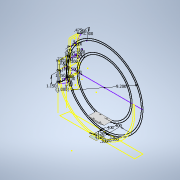
# Autodesk Inventor part: headband buffer
Saved by Autodesk Inventor 2022 (Build 260153000, 153)
## iProperties
Created: 2021-04-08
Part Number: headband buffer
Material: Generic
Document SubType Name: Modeling
Designer: chris
Density: 1 g/cm^3
Appearance: Default
Author: chris
Autodesk Inventor part; units mm, degrees
ref_plane "YZ Plane" through (0, 0, 0) normal (1, 0, 0) x (0, 1, 0)
ref_plane "XZ Plane" through (0, 0, 0) normal (0, 1, 0) x (-1, 0, 0)
ref_plane "XY Plane" through (0, 0, 0) normal (0, 0, 1) x (1, 0, 0)
sketch "Sketch1" plane through (0, 0, 0) normal (0, 0, 1) x (1, 0, 0)
  circle A0 centre (0, 0) radius 116.84
  circle A1 centre (0, 0) radius 111.76
  line L0 (-116.84, 0) -> (116.84, 0)
  circle A2 centre (0, 0) radius 78.74
  circle A3 centre (0, 0) radius 83.82
  point P0 (111.76, 0)
  point P1 (-111.76, 0)
  point P2 (-83.82, 0)
  point P3 (83.82, 0)
  point P4 (78.74, 0)
  point P5 (-78.74, 0)
  dimension "d0" = 233.68
  dimension "d1" = 5.08
  dimension "d45" = 38.1
  dimension "d46" = 5.08
  constraints: 4 centre point, 2 end point, 2 point on circle, 1 coincident, 1 horizontal
  measures "d0" diameter of A0
  measures "d1" radial gap between concentric circles of A0 A1
  measures "d45" radial gap between concentric circles of A0 A2
  measures "d46" radial gap between concentric circles of A2 A3
extrude "Extrusion1" add sketch "Sketch1" along normal blind 25.4 contours A0 L0 A1 picked at (7.308, -113.0578)
sketch "Sketch2" plane through (-116.84, 0, 0) normal (0, 1, 0) x (1, 0, 0)
  line L0 (5.08, 0) -> (0, 0) projected
  line L1 (0, 0) -> (0, -25.4) projected
  line L2 (5.08, -25.4) -> (0, -25.4) projected
  line L3 (5.08, 0) -> (5.08, -25.4) projected
  line L4 (233.68, 0) -> (228.6, 0) projected
  line L5 (228.6, 0) -> (228.6, -25.4) projected
  line L6 (233.68, -25.4) -> (228.6, -25.4) projected
  line L7 (233.68, 0) -> (233.68, -25.4) projected
  point P0 (116.84, 0)
extrude "Extrusion2" add sketch "Sketch2" along normal blind 25.4
sketch "Sketch3" plane through (-116.84, 0, 25.4) normal (-1, 0, 0) x (0, 0, 1)
  line L0 (-25.4, 0) -> (0, 0) projected
  line L1 (0, 0) -> (0, -34.29)
  line L2 (0, 0) -> (0, -111.76) projected
  line L3 (0, -34.29) -> (-25.4, -34.29)
  line L4 (-25.4, 0) -> (-25.4, -111.76) projected
  line L5 (-25.4, -34.29) -> (-25.4, 0)
  circle A0 centre (-5.7404, -2.54) radius 1.524
  circle A1 centre (-5.7404, -31.75) radius 1.524
  circle A2 centre (-19.6538, -2.54) radius 1.524
  circle A3 centre (-19.6538, -31.75) radius 1.524
  dimension "d6" = 34.29
  dimension "d7" = 3.048
  dimension "d8" = 3.048
  dimension "d9" = 3.048
  dimension "d10" = 3.048
  dimension "d11" = 29.21
  dimension "d12" = 2.54
  dimension "d13" = 5.7404
  constraints: 6 end point, 4 centre point, 2 horizontal alignment, 2 perpendicular, 2 point on line, 2 vertical alignment
  measures "d6" distance of L0.end L1.end
  measures "d7" diameter of A0
  measures "d8" diameter of A1
  measures "d9" diameter of A2
  measures "d10" diameter of A3
  measures "d11" distance of A1.centre A0.centre
  measures "d12" distance from line of L3 A1.centre
  measures "d13" distance from line of L1 A1.centre
extrude "Extrusion3" add sketch "Sketch3" against normal up to surface round surface about axis through (0, 0, 0) along (0, 0, 1) radius 116.84 far side no
extrude "Extrusion4" cut sketch "Sketch3" against normal blind 38.1 contours A0 | A1 | A2 | A3
sketch "Sketch4" plane through (-116.84, 25.4, 0) normal (-1, 0, 0) x (0, 0, 1)
  circle A0 centre (5.7462, -57.15) radius 1.524 projected
  circle A1 centre (5.7462, -27.94) radius 1.524 projected
  circle A2 centre (19.6596, -57.15) radius 1.524 projected
  circle A3 centre (19.6596, -27.94) radius 1.524 projected
  line L0 (25.4, -59.69) -> (25.4, 0) projected
  line L1 (0, 0) -> (25.4, 0) projected
  line L2 (0, -59.69) -> (0, 0) projected
  line L3 (0, -59.69) -> (25.4, -59.69) projected
  arc A4 (-7.874, -68.071) -> (0, -59.69) centre (-15.4136, -53.0981) ccw
  line L4 (-7.874, -68.071) -> (0, -71.373)
  line L5 (0, -25.4) -> (0, -137.16) projected
  line L6 (0, -71.373) -> (25.4, -59.69)
  arc A5 (0, -25.4) -> (-12.065, -6.604) centre (-32.1829, -32.7878) ccw
  line L7 (-12.065, -6.604) -> (0, 0)
  dimension "d22" = 16.764
  dimension "d23" = 33.02
  dimension "d24" = 6.604
  dimension "d25" = 12.065
  dimension "d26" = 7.874
  dimension "d27" = 3.302
  dimension "d28" = 25.4
  constraints: 6 end point, 4 point on circle, 2 centre point, 1 point on line
  measures "d22" radius of A4
  measures "d23" radius of A5
  measures "d24" vertical distance of L7.start L1.start
  measures "d25" horizontal distance of L1.start L7.start
  measures "d26" horizontal distance of L4.end L4.start
  measures "d27" vertical distance of L4.end L4.start
  measures "d28" horizontal distance of L0.start L4.end
extrude "Extrusion5" add sketch "Sketch4" against normal up to surface contours L6 L5 L3 | L5 L4 A4 round surface about axis through (0, 0, 0) along (0, 0, 1) radius 116.84 far side no
extrude "Extrusion6" add sketch "Sketch4" against normal up to surface (5.08 mm away) contours L2 A5 L7
sketch "Sketch5" plane through (116.84, 0, 0) normal (1, 0, 0) x (0, 0, -1)
  line L0 (0, 0) -> (-25.4, 0) projected
  line L1 (0, 0) -> (0, 25.4) projected
  line L2 (-25.4, 25.4) -> (0, 25.4) projected
  line L3 (-25.4, 0) -> (-25.4, 25.4) projected
  circle A0 centre (-12.7, 4.445) radius 1.524
  circle A1 centre (-12.7, 20.955) radius 1.524
  dimension "d29" = 3.048
  dimension "d30" = 3.048
  dimension "d31" = 4.445
  dimension "d32" = 4.445
  constraints: 2 centre point
  measures "d29" diameter of A0
  measures "d30" diameter of A1
  measures "d31" distance from line of L2 A1.centre
  measures "d32" distance from line of L0 A0.centre
extrude "Extrusion7" cut sketch "Sketch5" against normal blind 38.1 contours A0 | A1
sketch "Sketch6" plane through (0, 0, 25.4) normal (0, 0, 1) x (1, 0, 0)
  arc A0 (-111.76, 0) -> (111.76, 0) centre (0, 0) ccw projected
  line L0 (-111.76, 0) -> (-111.76, 25.4) projected
  line L1 (-116.84, 25.4) -> (-111.76, 25.4) projected
  line L2 (-116.84, -34.29) -> (-116.84, 25.4) projected
  line L3 (-116.84, -34.29) -> (-111.695, -34.29) projected
  arc A1 (-111.695, -34.29) -> (116.84, 0) centre (0, 0) ccw projected
  line L4 (116.84, 0) -> (116.84, 25.4) projected
  line L5 (111.76, 25.4) -> (116.84, 25.4) projected
  line L6 (111.76, 0) -> (111.76, 25.4) projected
  arc A2 (-107.4154, -45.973) -> (116.84, 0) centre (0, 0) ccw projected
  point P0 (0, -116.84)
  constraints: 1 point on circle
ref_plane "Work Plane1" through (0, -116.84, 25.4) normal (0, -1, 0) x (1, 0, 0)
sketch "Sketch7" plane through (0, -116.84, 25.4) normal (0, -1, 0) x (1, 0, 0)
  ellipse E0 centre (0, 74.5502) end of major axis (0, 328.573) minor radius 116.84 (-111.695, 0) -> (-107.4154, -25.4) ccw projected
  line L0 (-107.4154, -25.4) -> (116.84, -25.4) projected
  line L1 (116.84, -25.4) -> (116.84, 0) projected
  line L2 (-111.695, 0) -> (116.84, 0) projected
  circle A0 centre (10.16, -2.54) radius 1.524
  circle A1 centre (-10.16, -2.54) radius 1.524
  circle A2 centre (-10.16, -22.86) radius 1.524
  circle A3 centre (10.16, -22.86) radius 1.524
  point P0 (0, -25.4)
  dimension "d35" = 3.048
  dimension "d36" = 3.048
  dimension "d37" = 10.16
  dimension "d38" = 10.16
  dimension "d39" = 2.54
  dimension "d40" = 3.048
  dimension "d41" = 3.048
  dimension "d42" = 2.54
  constraints: 4 centre point, 2 horizontal alignment, 2 vertical alignment, 1 other
  measures "d35" diameter of A0
  measures "d36" diameter of A1
  measures "d37" horizontal distance of point (0, -25.4) A0.centre
  measures "d38" horizontal distance of point (0, -25.4) A1.centre
  measures "d39" distance from line of L2 A1.centre
  measures "d40" diameter of A2
  measures "d41" diameter of A3
  measures "d42" distance from line of L0 A3.centre
extrude "Extrusion8" cut sketch "Sketch7" against normal blind 38.1 contours A0 | A1 | A2 | A3
extrude "Extrusion9" add sketch "Sketch1" along normal blind 25.4 contours A3 L0 A2 picked at (6.1938, -80.0321)
sketch "Sketch8" plane through (78.74, 0, 0) normal (0, 1, 0) x (1, 0, 0)
  line L0 (5.08, 0) -> (0, 0) projected
  line L1 (0, 0) -> (0, -25.4) projected
  line L2 (5.08, -25.4) -> (0, -25.4) projected
  line L3 (5.08, 0) -> (5.08, -25.4) projected
  line L4 (-157.48, 0) -> (-162.56, 0) projected
  line L5 (-162.56, 0) -> (-162.56, -25.4) projected
  line L6 (-157.48, -25.4) -> (-162.56, -25.4) projected
  line L7 (-157.48, 0) -> (-157.48, -25.4) projected
  point P0 (-78.74, 0)
extrude "Extrusion10" add sketch "Sketch8" along normal blind 101.6
sketch "Sketch9" plane through (-83.82, 0, 25.4) normal (-1, 0, 0) x (0, 0, 1)
  point P0 (-25.4, 0)
sketch "Sketch10" plane through (-83.82, 0, 25.4) normal (-1, 0, 0) x (0, 0, 1)
  line L0 (-25.4, 0) -> (0, 0) projected
  line L1 (0, 0) -> (0, 101.6) projected
  line L2 (-25.4, 101.6) -> (0, 101.6) projected
  line L3 (-25.4, 0) -> (-25.4, 101.6) projected
  line L4 (-25.4, 0) -> (-25.4, 101.6) projected
  line L5 (-25.4, 101.6) -> (-37.465, 94.996)
  arc A0 (-25.4, 81.4487) -> (-37.465, 94.996) centre (-55.1426, 67.1065) ccw
  line L6 (-25.4, 33.6843) -> (-33.274, 36.9863)
  arc A1 (-33.274, 36.9863) -> (-25.4, 46.0711) centre (-41.1626, 51.7782) ccw
  line L7 (-25.4, 46.0711) -> (0, 46.0711)
  circle A2 centre (-19.6538, 48.6111) radius 1.524
  circle A3 centre (-19.6538, -31.75) radius 1.524 projected
  circle A4 centre (-19.6538, -2.54) radius 1.524 projected
  circle A5 centre (-5.7404, -31.75) radius 1.524 projected
  circle A6 centre (-5.7404, -2.54) radius 1.524 projected
  line L8 (0, -34.29) -> (0, 25.4) projected
  line L9 (-25.4, 25.4) -> (0, 25.4) projected
  line L10 (-25.4, 25.4) -> (-37.465, 18.796) projected
  arc A7 (-25.4, 0) -> (-37.465, 18.796) centre (-57.5829, -7.3878) ccw projected
  line L11 (-25.4, -34.29) -> (-25.4, 0) projected
  arc A8 (-33.274, -42.671) -> (-25.4, -34.29) centre (-40.8136, -27.6981) ccw projected
  line L12 (-33.274, -42.671) -> (-25.4, -45.973) projected
  line L13 (-25.4, -45.973) -> (0, -34.29) projected
  circle A9 centre (-5.7404, 48.6111) radius 1.524
  circle A10 centre (-5.7404, 77.8211) radius 1.524
  circle A11 centre (-19.6538, 77.8211) radius 1.524
  point P0 (-25.4, 81.4487)
  point P1 (-25.4, 46.0711)
  point P2 (-25.4, 46.0711)
  dimension "d51" = 12.065
  dimension "d52" = 6.604
  dimension "d53" = 33.02
  dimension "d54" = 3.302
  dimension "d55" = 7.874
  dimension "d56" = 16.764
  dimension "d57" = 3.048
  dimension "d58" = 2.54
  dimension "d59" = 3.048
  dimension "d60" = 3.048
  dimension "d61" = 3.048
  dimension "d62" = 29.21
  constraints: 6 centre point, 6 end point, 4 point on circle, 4 point on line, 2 vertical alignment, 1 horizontal alignment, 1 perpendicular
  measures "d51" distance from line of L3 L5.end
  measures "d52" vertical distance of L5.end L2.start
  measures "d53" radius of A0
  measures "d54" vertical distance of L6.start L6.end
  measures "d55" horizontal distance of L6.end L6.start
  measures "d56" radius of A1
  measures "d57" diameter of A2
  measures "d58" distance from line of L7 A2.centre
  measures "d59" diameter of A9
  measures "d60" diameter of A10
  measures "d61" diameter of A11
  measures "d62" distance of A9.centre A10.centre
extrude "Extrusion11" cut sketch "Sketch10" against normal blind 76.2 contours A2 | A9 | A10 | A11
extrude "Extrusion12" add sketch "Sketch10" against normal blind 5.08 contours L6 A1 L3 | A0 L5 L3
extrude "Extrusion13" cut sketch "Sketch7" against normal blind 736.6 contours A0 | A1 | A2 | A3
sketch "Sketch11" plane through (83.82, 0, 0) normal (1, 0, 0) x (0, 0, -1)
  circle A0 centre (-12.7, 97.155) radius 1.524
  line L0 (-25.4, 101.6) -> (0, 101.6) projected
  circle A1 centre (-12.7, 80.645) radius 1.524
  circle A2 centre (-12.7, 20.955) radius 1.524 projected
  circle A3 centre (-12.7, 4.445) radius 1.524 projected
  line L1 (0, 0) -> (-25.4, 0) projected
  line L2 (0, 0) -> (0, 25.4) projected
  line L3 (-25.4, 25.4) -> (0, 25.4) projected
  line L4 (-25.4, 0) -> (-25.4, 25.4) projected
  dimension "d69" = 3.048
  dimension "d70" = 4.445
  dimension "d71" = 3.048
  dimension "d72" = 16.51
  constraints: 2 centre point
  measures "d69" diameter of A0
  measures "d70" distance from line of L0 A0.centre
  measures "d71" diameter of A1
  measures "d72" distance of A0.centre A1.centre
extrude "Extrusion14" cut sketch "Sketch11" against normal blind 50.8 contours A0 | A1
sketch "Sketch12" plane through (0, 0, 25.4) normal (0, 0, 1) x (1, 0, 0)
  line L0 (93.2963, 11.7206) -> (81.9248, -56.1526)
  line L1 (81.9248, -56.1526) -> (43.191, -89.9115)
  line L2 (43.191, -89.9115) -> (-42.0947, -94.5311)
  line L3 (-42.0947, -94.5311) -> (-91.8447, -45.4919)
  line L4 (-91.8447, -45.4919) -> (-123.4714, 72.4866)
  line L5 (-123.4714, 72.4866) -> (-141.5946, -65.0365)
  line L6 (-141.5946, -65.0365) -> (-46.7143, -147.8346)
  line L7 (-46.7143, -147.8346) -> (105.023, -111.9436)
  line L8 (105.023, -111.9436) -> (135.128, -5.6052)
  line L9 (135.128, -5.6052) -> (115.3284, 89.5437)
  line L10 (115.3284, 89.5437) -> (93.2963, 11.7206)
  point P0 (0, 0)
  constraints: 22 end point, 1 parallel
extrude "Extrusion15" cut sketch "Sketch12" against normal blind 50.8
sketch "Sketch13" plane through (0, 0, 0) normal (0, 0, -1) x (-1, 0, 0)
  line L0 (83.82, 101.6) -> (83.82, 94.996) projected
  line L1 (78.74, 101.6) -> (83.82, 101.6) projected
  line L2 (78.74, 94.996) -> (78.74, 101.6) projected
  line L3 (83.82, 94.996) -> (78.74, 94.996) projected
  line L4 (78.74, 81.4487) -> (78.74, 94.996) projected
  line L5 (83.82, 94.996) -> (83.82, 81.4487) projected
  line L6 (83.82, 94.996) -> (78.74, 94.996) projected
  line L7 (78.74, 81.4487) -> (78.74, 94.996) projected
  line L8 (83.82, 81.4487) -> (78.74, 81.4487) projected
  line L9 (83.82, 81.4487) -> (78.74, 81.4487) projected
  line L10 (78.74, 46.0711) -> (78.74, 81.4487) projected
  line L11 (78.74, 46.0711) -> (83.82, 46.0711) projected
  line L12 (83.82, 46.0711) -> (83.82, 81.4487) projected
  line L13 (83.82, 46.0711) -> (83.82, 36.9863) projected
  line L14 (78.74, 46.0711) -> (83.82, 46.0711) projected
  line L15 (78.74, 36.9863) -> (78.74, 46.0711) projected
  line L16 (83.82, 36.9863) -> (78.74, 36.9863) projected
  line L17 (83.82, 36.9863) -> (83.82, 33.6843) projected
  line L18 (83.82, 36.9863) -> (78.74, 36.9863) projected
  line L19 (78.74, 33.6843) -> (78.74, 36.9863) projected
  line L20 (83.82, 33.6843) -> (78.74, 33.6843) projected
  point P0 (0, 0)
extrude "Extrusion16" cut sketch "Sketch13" along normal blind 25.4
sketch "Sketch14" plane through (-78.74, 0, 0) normal (1, 0, 0) x (0, 0, -1)
  circle A0 centre (-19.6596, 48.6111) radius 1.524 projected
  line L0 (-19.6596, 48.6111) -> (-19.6596, 26.6111)
  circle A1 centre (-19.6596, 26.6111) radius 1.524
  line L1 (-5.7521, 48.6111) -> (-5.7521, 26.6111)
  circle A2 centre (-5.7521, 26.6111) radius 1.524
  line L2 (-19.6596, 26.6111) -> (-19.6596, -2.5989)
  circle A3 centre (-19.6596, -2.5989) radius 1.524
  circle A4 centre (-5.7521, -2.5989) radius 1.524
  point P0 (0, 0)
  dimension "d79" = 22
  dimension "d80" = 3.048
  dimension "d81" = 3.048
  dimension "d82" = 29.21
  dimension "d83" = 3.048
  dimension "d84" = 3.048
  constraints: 6 end point, 4 centre point, 3 coincident, 3 vertical
  measures "d79" distance of L0.start L0.end
  measures "d80" diameter of A1
  measures "d81" diameter of A2
  measures "d82" distance of L2.start L2.end
  measures "d83" diameter of A3
  measures "d84" diameter of A4
extrude "Extrusion17" cut sketch "Sketch14" along normal mid plane 50.8 contours A1 L2 L0 | L0 L2 A1 | A2 | A3 | A4
sketch "Sketch15" plane through (-78.74, 0, 0) normal (1, 0, 0) x (0, 0, -1)
  circle A0 centre (-12.7, 97.155) radius 1.524 projected
  circle A1 centre (-12.7, 80.645) radius 1.524 projected
  line L0 (0, 0) -> (-25.4, 0) projected
  line L1 (0, 0) -> (0, 101.6) projected
  line L2 (-25.4, 101.6) -> (0, 101.6) projected
  line L3 (-25.4, 0) -> (-25.4, 101.6) projected
extrude "Extrusion18" add sketch "Sketch10" against normal up to surface (5.08 mm away) contours L7 L3 L2 L1 | A2 | A9 | A10 | A11
sketch "Sketch16" plane through (0, -116.84, 25.4) normal (0, -1, 0) x (1, 0, 0)
  spline S0 degree 7 poles (-8.636, -22.86) (-8.636, -22.6774) (-8.6615, -22.4948) (-8.7126, -22.3146) (-8.7898, -22.1394) (-8.8943, -21.9728) (-9.0271, -21.8194) (-9.3317, -21.5673) (-9.5016, -21.461) (-9.6948, -21.3783) (-9.9044, -21.3271) (-10.1213, -21.3114) (-10.3357, -21.3317) (-10.746, -21.437) (-10.9352, -21.5217) (-11.1032, -21.6313) (-11.2479, -21.7601) (-11.3686, -21.9029) (-11.4653, -22.0547) (-11.6272, -22.3986) (-11.6844, -22.5974) (-11.7102, -22.8026) (-11.7042, -23.0098) (-11.6661, -23.2142) (-11.5963, -23.4109) (-11.4178, -23.7355) (-11.3202, -23.8718) (-11.202, -23.9993) (-11.0634, -24.114) (-10.9053, -24.2115) (-10.7296, -24.2872) (-10.3508, -24.3844) (-10.1525, -24.4055) (-9.9512, -24.3959) (-9.7549, -24.3553) (-9.5712, -24.2867) (-9.4065, -24.1963) (-9.0805, -23.9595) (-8.9294, -23.8009) (-8.8106, -23.6259) (-8.7228, -23.4405) (-8.6649, -23.2488) (-8.636, -23.0544) (-8.636, -22.86) knots 0 0 0 0 0 0 0 0 0.15177 0.15177 0.15177 0.15177 0.15177 0.15177 0.286279 0.286279 0.286279 0.286279 0.286279 0.286279 0.423214 0.423214 0.423214 0.423214 0.423214 0.423214 0.587338 0.587338 0.587338 0.587338 0.587338 0.587338 0.713828 0.713828 0.713828 0.713828 0.713828 0.713828 0.838738 0.838738 0.838738 0.838738 0.838738 0.838738 1 1 1 1 1 1 1 1 projected
  spline S1 degree 7 poles (11.684, -2.54) (11.684, -2.3573) (11.6584, -2.1745) (11.6073, -1.9942) (11.53, -1.819) (11.4254, -1.6525) (11.2928, -1.4992) (10.9884, -1.2474) (10.8188, -1.1413) (10.6258, -1.0586) (10.4164, -1.0073) (10.1996, -0.9914) (9.9849, -1.0115) (9.574, -1.117) (9.3847, -1.2017) (9.2167, -1.3114) (9.0719, -1.4403) (8.9512, -1.5831) (8.8546, -1.7349) (8.6927, -2.0789) (8.6356, -2.2776) (8.6099, -2.4826) (8.6158, -2.6896) (8.6538, -2.8939) (8.7236, -3.0907) (8.9021, -3.4153) (8.9997, -3.5516) (9.1179, -3.6792) (9.2565, -3.7939) (9.4146, -3.8915) (9.5904, -3.9672) (9.9697, -4.0646) (10.1682, -4.0856) (10.3696, -4.0757) (10.5658, -4.0351) (10.7492, -3.9665) (10.9137, -3.8762) (11.2392, -3.6397) (11.3903, -3.4812) (11.5092, -3.3064) (11.597, -3.1209) (11.655, -2.9292) (11.684, -2.7345) (11.684, -2.54) knots 0 0 0 0 0 0 0 0 0.15183 0.15183 0.15183 0.15183 0.15183 0.15183 0.286406 0.286406 0.286406 0.286406 0.286406 0.286406 0.423049 0.423049 0.423049 0.423049 0.423049 0.423049 0.587262 0.587262 0.587262 0.587262 0.587262 0.587262 0.713539 0.713539 0.713539 0.713539 0.713539 0.713539 0.838569 0.838569 0.838569 0.838569 0.838569 0.838569 1 1 1 1 1 1 1 1 projected
  spline S2 degree 7 poles (11.684, -22.86) (11.684, -22.6773) (11.6584, -22.4945) (11.6073, -22.3142) (11.53, -22.139) (11.4254, -21.9725) (11.2928, -21.8192) (10.9884, -21.5674) (10.8188, -21.4613) (10.6258, -21.3786) (10.4164, -21.3273) (10.1996, -21.3114) (9.9849, -21.3315) (9.574, -21.437) (9.3847, -21.5217) (9.2167, -21.6314) (9.0719, -21.7603) (8.9512, -21.9031) (8.8546, -22.0549) (8.6927, -22.3989) (8.6356, -22.5976) (8.6099, -22.8026) (8.6158, -23.0096) (8.6538, -23.2139) (8.7236, -23.4107) (8.9021, -23.7353) (8.9997, -23.8716) (9.1179, -23.9992) (9.2565, -24.1139) (9.4146, -24.2115) (9.5904, -24.2872) (9.9697, -24.3846) (10.1682, -24.4056) (10.3696, -24.3957) (10.5658, -24.3551) (10.7492, -24.2865) (10.9137, -24.1962) (11.2392, -23.9597) (11.3903, -23.8012) (11.5092, -23.6264) (11.597, -23.4409) (11.655, -23.2492) (11.684, -23.0545) (11.684, -22.86) knots 0 0 0 0 0 0 0 0 0.15183 0.15183 0.15183 0.15183 0.15183 0.15183 0.286406 0.286406 0.286406 0.286406 0.286406 0.286406 0.423049 0.423049 0.423049 0.423049 0.423049 0.423049 0.587262 0.587262 0.587262 0.587262 0.587262 0.587262 0.713539 0.713539 0.713539 0.713539 0.713539 0.713539 0.838569 0.838569 0.838569 0.838569 0.838569 0.838569 1 1 1 1 1 1 1 1 projected
  spline S3 degree 7 poles (-8.636, -2.54) (-8.636, -2.3574) (-8.6615, -2.1748) (-8.7126, -1.9946) (-8.7898, -1.8194) (-8.8943, -1.6528) (-9.0271, -1.4994) (-9.3317, -1.2473) (-9.5016, -1.141) (-9.6948, -1.0583) (-9.9044, -1.0071) (-10.1213, -0.9914) (-10.3357, -1.0117) (-10.746, -1.117) (-10.9352, -1.2017) (-11.1032, -1.3113) (-11.2479, -1.4401) (-11.3686, -1.5829) (-11.4653, -1.7347) (-11.6272, -2.0786) (-11.6844, -2.2774) (-11.7102, -2.4826) (-11.7042, -2.6898) (-11.6661, -2.8942) (-11.5963, -3.0909) (-11.4178, -3.4155) (-11.3202, -3.5518) (-11.202, -3.6793) (-11.0634, -3.794) (-10.9053, -3.8915) (-10.7296, -3.9672) (-10.3508, -4.0644) (-10.1525, -4.0855) (-9.9512, -4.0759) (-9.7549, -4.0353) (-9.5712, -3.9667) (-9.4065, -3.8763) (-9.0805, -3.6395) (-8.9294, -3.4809) (-8.8106, -3.3059) (-8.7228, -3.1205) (-8.6649, -2.9288) (-8.636, -2.7344) (-8.636, -2.54) knots 0 0 0 0 0 0 0 0 0.15177 0.15177 0.15177 0.15177 0.15177 0.15177 0.286279 0.286279 0.286279 0.286279 0.286279 0.286279 0.423214 0.423214 0.423214 0.423214 0.423214 0.423214 0.587338 0.587338 0.587338 0.587338 0.587338 0.587338 0.713828 0.713828 0.713828 0.713828 0.713828 0.713828 0.838738 0.838738 0.838738 0.838738 0.838738 0.838738 1 1 1 1 1 1 1 1 projected
  line L0 (-83.82, -25.4) -> (83.82, -25.4) projected
  line L1 (83.82, -25.4) -> (83.82, 0) projected
  line L2 (-83.82, 0) -> (83.82, 0) projected
  line L3 (-83.82, -25.4) -> (-83.82, 0) projected
  circle A0 centre (-10.16, -2.54) radius 1.524 projected
  point P0 (0, -25.4)
  constraints: 1 horizontal alignment, 6 other
sketch "Sketch17" plane through (0, 0, 0) normal (0, 0, -1) x (-1, 0, 0)
  line L0 (-43.1955, -53.5651) -> (6.3345, -53.5651)
  arc A0 (-78.74, 0) -> (78.74, 0) centre (0, 0) ccw projected
  line L1 (-24.765, -74.7441) -> (24.765, -74.7441)
  dimension "d89" = 49.53
  dimension "d90" = 49.53
  constraints: 4 end point, 2 horizontal, 2 point on circle
  measures "d89" distance of L0.start L0.end
  measures "d90" distance of L1.start L1.end
extrude "Extrusion19" add sketch "Sketch17" against normal up to surface (25.4 mm away)
extrude "Extrusion20" cut sketch "Sketch16" against normal through all contours S0 | S1 | S2 | S3
sketch "Sketch18" plane through (0, 0, 0) normal (0, 0, -1) x (-1, 0, 0)
  circle A0 centre (0, 0) radius 78.74 projected
  circle A1 centre (0, 0) radius 83.82 projected
  line L0 (-78.74, 0) -> (-78.74, 101.6) projected
  line L1 (-83.82, 0) -> (-83.82, 101.6) projected
  line L2 (-83.82, 101.6) -> (-78.74, 101.6) projected
  line L3 (78.74, 0) -> (78.74, 101.6) projected
  line L4 (83.82, 0) -> (83.82, 101.6) projected
  line L5 (78.74, 101.6) -> (83.82, 101.6) projected
extrude "Extrusion21" cut sketch "Sketch18" against normal through all contours L3 A1 L0 A0 | L3 L5 L4 A1 | A1 L1 L2 L0 picked at (-79.6765, 16.0382)
body "Solid1"
